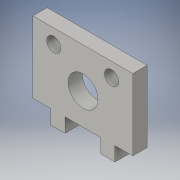
# Autodesk Inventor part: Near Holder
Saved by Autodesk Inventor 2016 (Build 200138000, 138)
## iProperties
Created: 2016-04-25
Part Number: Near Holder
Material: Generic
Document SubType Name: Modeling
Designer: rubenjm
Density: 1 g/cm^3
Appearance: Default
Author: rubenjm
Autodesk Inventor part; units mm, degrees
ref_plane "YZ Plane" through (0, 0, 0) normal (1, 0, 0) x (0, 1, 0)
ref_plane "XZ Plane" through (0, 0, 0) normal (0, 1, 0) x (-1, 0, 0)
ref_plane "XY Plane" through (0, 0, 0) normal (0, 0, 1) x (1, 0, 0)
sketch "Sketch1" plane through (0, 0, 0) normal (0, 0, 1) x (1, 0, 0)
  circle A0 centre (44.6106, 27.94) radius 6.985 construction
  circle A1 centre (18.5683, 50.8) radius 6.35 construction
  line L0 (0, 63.5) -> (0, 50.8) construction
  line L1 (0, 50.8) -> (12.7, 50.8) construction
  line L2 (12.7, 50.8) -> (12.7, 63.5) construction
  line L3 (12.7, 63.5) -> (0, 63.5) construction
  circle A2 centre (70.0106, 50.8) radius 6.35 construction
  line L4 (31.779, 27.94) -> (38.1948, 39.0525) construction
  line L5 (38.1948, 39.0525) -> (51.0264, 39.0525) construction
  line L6 (51.0264, 39.0525) -> (57.4422, 27.94) construction
  line L7 (57.4422, 27.94) -> (51.0264, 16.8275) construction
  line L8 (51.0264, 16.8275) -> (38.1948, 16.8275) construction
  line L9 (0, 63.5) -> (0, 0)
  line L10 (88.9, 0) -> (88.9, 63.5)
  line L11 (88.9, 63.5) -> (0, 63.5)
  line L12 (44.45, 0) -> (44.45, 27.94) construction
  line L13 (44.45, 0) -> (44.45, 27.94) construction
  line L14 (31.779, 27.94) -> (38.1948, 16.8275) construction
  line L15 (44.45, 0) -> (44.45, 63.5) construction
  line L16 (44.45, 0) -> (60.325, 0) construction
  line L17 (44.45, 0) -> (44.45, 15.875) construction
  line L18 (60.325, 0) -> (60.325, -12.7)
  line L19 (60.325, -12.7) -> (73.025, -12.7)
  line L20 (73.025, -12.7) -> (73.025, 0)
  line L21 (44.45, 0) -> (28.575, 0) construction
  line L22 (28.575, 0) -> (28.575, -12.7)
  line L23 (15.875, -12.7) -> (15.875, 0)
  line L24 (28.575, -12.7) -> (15.875, -12.7)
  line L25 (0, 0) -> (15.875, 0)
  line L26 (28.575, 0) -> (60.325, 0)
  line L27 (73.025, 0) -> (88.9, 0)
  point P0 (0, 0)
  point P1 (0, 0)
  point P2 (12.8606, 0)
  dimension "d0" = 88.9
  dimension "d1" = 63.5
  dimension "d2" = 15.875
  dimension "d3" = 90
  dimension "d4" = 12.7
  dimension "d5" = 12.7
  constraints: 56 end point, 7 parallel, 5 perpendicular, 4 symmetric about line, 3 centre point, 3 midpoint, 2 equal length, 1 point on line
  measures "d0" distance of L10.end L0.start
  measures "d1" distance of L10.start L10.end
  measures "d2" distance of L15.start L16.end
  measures "d3" angle of L16 L17
  measures "d4" distance of L20.end L19.end
  measures "d5" distance of L19.end L18.end
extrude "Extrusion1" add sketch "Sketch1" along normal blind 12.7
sketch "Sketch2" plane through (0, 0, 12.7) normal (0, 0, 1) x (1, 0, 0)
  circle A0 centre (18.5683, 50.8) radius 6.35
  line L0 (12.7, 50.8) -> (12.7, 63.5) construction
  line L1 (0, 50.8) -> (12.7, 50.8) construction
  line L2 (31.779, 27.94) -> (38.1948, 39.0525) construction
  line L3 (44.45, 0) -> (44.45, 15.875) construction
  line L4 (38.1948, 39.0525) -> (51.0264, 39.0525) construction
  line L5 (51.0264, 16.8275) -> (38.1948, 16.8275) construction
  circle A1 centre (44.6106, 27.94) radius 13.335
  line L6 (51.0264, 39.0525) -> (57.4422, 27.94) construction
  line L7 (57.4422, 27.94) -> (51.0264, 16.8275) construction
  circle A2 centre (70.0106, 50.8) radius 6.35
  line L8 (44.45, 0) -> (44.45, 27.94) construction
  line L9 (31.779, 27.94) -> (38.1948, 16.8275) construction
  line L10 (44.45, 0) -> (44.45, 27.94) construction
  line L11 (88.9, 0) -> (88.9, 63.5) construction
  line L12 (0, 0) -> (88.9, 0) construction
  line L13 (28.575, 0) -> (60.325, 0) construction
  line L14 (44.45, 0) -> (44.45, 63.5) construction
  line L15 (88.9, 63.5) -> (0, 63.5) construction
  line L16 (0, 63.5) -> (0, 0) projected
  dimension "d8" = 26.67
  dimension "d9" = 12.7
  dimension "d10" = 12.7
  dimension "d11" = 18.5683
  dimension "d12" = 12.7
  dimension "d13" = 18.8894
  dimension "d14" = 12.7
  dimension "d15" = 25.8817
  dimension "d16" = 25.5606
  dimension "d17" = 27.94
  dimension "d18" = 44.45
  constraints: 32 end point, 3 centre point, 2 midpoint, 1 collinear, 1 horizontal, 1 point on line
  measures "d8" diameter of A1
  measures "d9" diameter of A0
  measures "d10" diameter of A2
  measures "d11" distance from line of L16 A0.centre
  measures "d12" distance from line of L15 A0.centre
  measures "d13" distance from line of L11 A2.centre
  measures "d14" distance from line of L15 A2.centre
  measures "d15" distance from line of L14 A0.centre
  measures "d16" distance from line of L14 A2.centre
  measures "d17" vertical distance of L3.start A1.centre
  measures "d18" distance from line of L16 L10.end
extrude "Extrusion2" cut sketch "Sketch2" against normal blind 12.7
body "Solid1"
